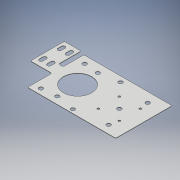
# Autodesk Inventor part: piezaaa
Saved by Autodesk Inventor 2018 (Build 220112000, 112)
## iProperties
Created: 2018-10-04
Part Number: piezaaa
Material: Genérico
Document SubType Name: Modeling
Designer: Vayron
Density: 1 g/cm^3
Appearance: Valor por defecto
Author: Vayron
Autodesk Inventor part; units mm, degrees
ref_plane "YZ Plane" through (0, 0, 0) normal (1, 0, 0) x (0, 1, 0)
ref_plane "XZ Plane" through (0, 0, 0) normal (0, 1, 0) x (-1, 0, 0)
ref_plane "XY Plane" through (0, 0, 0) normal (0, 0, 1) x (1, 0, 0)
sketch "Boceto1" plane through (0, 0, 0) normal (0, 0, 1) x (1, 0, 0)
  line L0 (-122.755, 65.145) -> (122.755, -65.145) construction
  line L1 (122.755, 65.145) -> (-122.755, -65.145) construction
  line L2 (-122.755, 65.145) -> (-85.295, 65.145)
  line L3 (-122.755, 65.145) -> (-122.755, -10.585)
  line L4 (-85.295, 65.145) -> (-85.295, 14.655)
  line L5 (-85.295, 14.655) -> (-74.705, 14.655)
  line L6 (-74.705, 14.655) -> (-74.705, 61.075)
  line L7 (-74.705, 61.075) -> (122.755, 61.075)
  line L8 (-122.755, -10.585) -> (-74.705, -10.585)
  line L9 (-74.705, -10.585) -> (-74.705, -65.145)
  line L10 (-74.705, -65.145) -> (122.755, -65.145)
  line L11 (122.755, 61.075) -> (122.755, -65.145)
  line L12 (122.755, 61.075) -> (122.755, -4.07)
  circle A0 centre (93.325, -27.57) radius 2.5
  circle A1 centre (93.325, 19.43) radius 2.5
  circle A2 centre (46.325, 19.43) radius 2.5
  circle A3 centre (46.325, -27.57) radius 2.5
  line L13 (122.755, 61.075) -> (122.755, -4.07)
  line L14 (122.755, 61.075) -> (122.755, -4.07)
  line L15 (122.755, 61.075) -> (122.755, -4.07)
  circle A4 centre (69.825, -4.07) radius 4.5
  circle A5 centre (90.185, 39.09) radius 4.5
  circle A6 centre (88.9646, -47.2127) radius 4.5
  circle A7 centre (19.745, 48.86) radius 4.5
  circle A8 centre (-56.385, 44.38) radius 4.5
  circle A9 centre (-57.6054, -52.5027) radius 4.5
  circle A10 centre (18.5246, -56.9827) radius 4.5
  circle A11 centre (-23.815, 41.325) radius 4.5
  circle A12 centre (-23.815, -49.465) radius 4.5
  circle A13 centre (-23.815, -4.07) radius 31.755
  line L16 (-116.6465, 10.975) -> (-116.6465, 2.875)
  line L17 (-108.5035, 2.875) -> (-108.5035, 10.975)
  arc A14 (-108.5035, 10.975) -> (-116.6465, 10.975) centre (-112.575, 10.975) ccw
  arc A15 (-116.6465, 2.875) -> (-108.5035, 2.875) centre (-112.575, 2.875) ccw
  line L18 (-98.7365, 10.975) -> (-98.7365, 2.875)
  line L19 (-90.5935, 2.875) -> (-90.5935, 10.975)
  arc A16 (-90.5935, 10.975) -> (-98.7365, 10.975) centre (-94.665, 10.975) ccw
  arc A17 (-98.7365, 2.875) -> (-90.5935, 2.875) centre (-94.665, 2.875) ccw
  line L20 (-116.6465, 52.505) -> (-116.6465, 44.405)
  line L21 (-108.5035, 44.405) -> (-108.5035, 52.505)
  line L22 (-90.5935, 52.505) -> (-90.5935, 44.405)
  line L23 (-98.7365, 44.405) -> (-98.7365, 52.505)
  arc A18 (-108.5035, 52.505) -> (-116.6465, 52.505) centre (-112.575, 52.505) ccw
  arc A19 (-116.6465, 44.405) -> (-108.5035, 44.405) centre (-112.575, 44.405) ccw
  arc A20 (-98.7365, 44.405) -> (-90.5935, 44.405) centre (-94.665, 44.405) ccw
  arc A21 (-90.5935, 52.505) -> (-98.7365, 52.505) centre (-94.665, 52.505) ccw
  point P0 (0, 0)
  point P1 (-112.575, 65.145)
  point P2 (-94.665, 65.145)
  dimension "d0" = 245.51
  dimension "d1" = 130.29
  dimension "d2" = 37.46
  dimension "d3" = 75.73
  dimension "d18" = 5
  dimension "d19" = 5
  dimension "d20" = 5
  dimension "d21" = 5
  dimension "d27" = 9
  dimension "d28" = 9
  dimension "d29" = 9
  dimension "d34" = 9
  dimension "d35" = 9
  dimension "d40" = 9
  dimension "d41" = 9
  dimension "d45" = 9
  dimension "d46" = 9
  dimension "d47" = 63.51
  constraints: 48 end point, 22 centre point, 16 point on circle, 8 tangent, 6 parallel, 5 point on line, 5 vertical, 3 collinear, 2 midpoint, 2 perpendicular
  measures "d0" distance of L0.end L1.end
  measures "d1" distance of L1.start L0.end
  measures "d2" distance of L0.start L2.end
  measures "d3" distance of L0.start L3.end
  measures "d18" diameter of A0
  measures "d19" diameter of A1
  measures "d20" diameter of A2
  measures "d21" diameter of A3
  measures "d27" diameter of A4
  measures "d28" diameter of A5
  measures "d29" diameter of A6
  measures "d34" diameter of A7
  measures "d35" diameter of A8
  measures "d40" diameter of A9
  measures "d41" diameter of A10
  measures "d45" diameter of A11
  measures "d46" diameter of A12
  measures "d47" diameter of A13
extrude "Extrusión2" add sketch "Boceto1" along normal mid plane 0.8
fillet "Empalme2" radius 3 10 edges at (-85.295, 14.655, 0) (-74.705, 14.655, 0) (-85.295, 65.145, 0) (-122.755, 65.145, 0) (-74.705, 61.075, 0) (122.755, 61.075, 0) (122.755, -65.145, 0) (-74.705, -65.145, 0) (-74.705, -10.585, 0) (-122.755, -10.585, 0)
